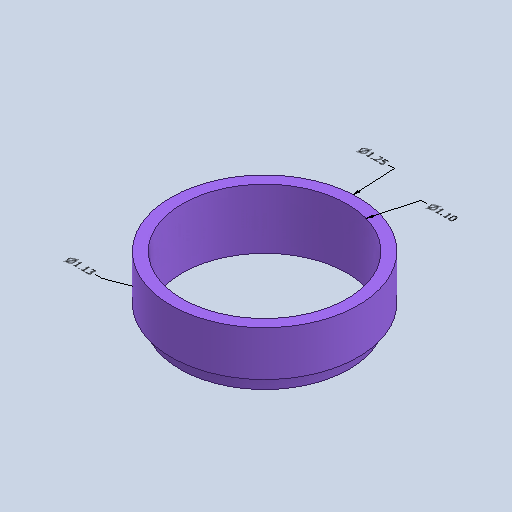
# Autodesk Inventor part: simulatedFilterWithoutThreads
Saved by Autodesk Inventor 2022.1 (Build 261234000, 234)
## iProperties
Created: 2020-09-08
Part Number: simulatedFilterWithoutThreads
Material: PBT Plastic
Document SubType Name: Modeling
Designer: robst
Density: 1.31 g/cm^3
Appearance: Violet
Author: robst
Autodesk Inventor part; units mm, degrees
ref_plane "YZ Plane" through (0, 0, 0) normal (1, 0, 0) x (0, 1, 0)
ref_plane "XZ Plane" through (0, 0, 0) normal (0, 1, 0) x (-1, 0, 0)
ref_plane "XY Plane" through (0, 0, 0) normal (0, 0, 1) x (1, 0, 0)
sketch "Sketch1" plane through (0, 0, 0) normal (0, 0, 1) x (1, 0, 0)
  line L0 (-14.351, 0) -> (-14.351, 2.54)
  line L1 (-14.351, 2.54) -> (-15.875, 2.54)
  line L2 (-15.875, 2.54) -> (-15.875, 10.16)
  line L3 (-15.875, 10.16) -> (-13.97, 10.16)
  line L4 (-13.97, 10.16) -> (-13.97, 0)
  line L5 (-13.97, 0) -> (-14.351, 0)
  line L6 (0, -2.032) -> (0, 12.192) projected
  point P0 (0, 0)
  dimension "d0" = 2.54
  dimension "d1" = 7.62
  dimension "d2" = 13.97
  dimension "d3" = 15.875
  dimension "d4" = 14.351
  constraints: 12 end point, 5 perpendicular, 1 vertical
  measures "d0" distance of L0.start L0.end
  measures "d1" distance of L1.end L2.end
  measures "d2" distance from line of L4 point (0, 0)
  measures "d3" distance from line of L2 point (0, 0)
  measures "d4" distance from line of L0 point (0, 0)
revolve "Revolution1" add sketch "Sketch1" angle 360 about axis through (0, -10, 0) along (0, 1, 0)
equation "\"d0\" = shortHeight"
equation "\"d1\" = tallHeight"
equation "\"d3\" = largeExteriorRadius"
equation "\"d4\" = smallerExteriorRadius"
equation "\"largeExteriorDiameter\" = 31.75"
equation "\"smallerExteriorDiameter\" = 28.702"
equation "\"shortHeight\" = 2.54"
equation "\"largeExteriorRadius\" = 0.5 * largeExteriorDiameter"
equation "\"smallerExteriorRadius\" = 0.5 * smallerExteriorDiameter"
equation "\"tallHeight\" = 7.62"
body "Solid1"
